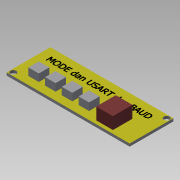
# Autodesk Inventor part: mode
Saved by Autodesk Inventor 2015 SP1 (Build 190203100, 203)
## iProperties
Created: 2015-01-28
Part Number: mode
Material: Generic
Document SubType Name: Modeling
Designer: Rafi Kurnia Putra
Density: 1 g/cm^3
Appearance: Default
Author: Rafi Kurnia Putra
Autodesk Inventor part; units mm, degrees
ref_plane "YZ Plane" through (0, 0, 0) normal (1, 0, 0) x (0, 1, 0)
ref_plane "XZ Plane" through (0, 0, 0) normal (0, 1, 0) x (-1, 0, 0)
ref_plane "XY Plane" through (0, 0, 0) normal (0, 0, 1) x (1, 0, 0)
sketch "Sketch1" plane through (0, 0, 0) normal (0, 1, 0) x (-1, 0, 0)
  line L0 (36.775, 13.07) -> (-36.775, 13.07)
  line L1 (-36.775, 13.07) -> (-36.775, -13.07)
  line L2 (-36.775, -13.07) -> (36.775, -13.07)
  line L3 (36.775, -13.07) -> (36.775, 13.07)
  line L4 (36.775, 13.07) -> (-36.775, -13.07) construction
  line L5 (-36.775, 13.07) -> (36.775, -13.07) construction
  circle A0 centre (-34.775, -11.07) radius 1.75
  circle A1 centre (34.775, 11.07) radius 1.75
  line L6 (-14.775, -0.61) -> (-24.775, -0.61)
  line L7 (-24.775, -0.61) -> (-24.775, 11.07)
  line L8 (-24.775, 11.07) -> (-14.775, 11.07)
  line L9 (-14.775, 11.07) -> (-14.775, -0.61)
  line L10 (-14.775, -0.61) -> (-24.775, 11.07) construction
  line L11 (-24.775, -0.61) -> (-14.775, 11.07) construction
  line L12 (28.4695, 2.1) -> (22.2095, 2.1)
  line L13 (22.2095, 2.1) -> (22.2095, 8.36)
  line L14 (22.2095, 8.36) -> (28.4695, 8.36)
  line L15 (28.4695, 8.36) -> (28.4695, 2.1)
  line L16 (28.4695, 2.1) -> (22.2095, 8.36) construction
  line L17 (22.2095, 2.1) -> (28.4695, 8.36) construction
  line L18 (18.4695, 8.36) -> (12.2095, 8.36)
  line L19 (12.2095, 8.36) -> (12.2095, 2.1)
  line L20 (12.2095, 2.1) -> (18.4695, 2.1)
  line L21 (18.4695, 2.1) -> (18.4695, 8.36)
  line L22 (18.4695, 8.36) -> (12.2095, 2.1) construction
  line L23 (12.2095, 8.36) -> (18.4695, 2.1) construction
  line L24 (8.4695, 8.36) -> (2.2095, 8.36)
  line L25 (2.2095, 8.36) -> (2.2095, 2.1)
  line L26 (2.2095, 2.1) -> (8.4695, 2.1)
  line L27 (8.4695, 2.1) -> (8.4695, 8.36)
  line L28 (8.4695, 8.36) -> (2.2095, 2.1) construction
  line L29 (2.2095, 8.36) -> (8.4695, 2.1) construction
  line L30 (-1.5305, 8.36) -> (-7.7905, 8.36)
  line L31 (-7.7905, 8.36) -> (-7.7905, 2.1)
  line L32 (-7.7905, 2.1) -> (-1.5305, 2.1)
  line L33 (-1.5305, 2.1) -> (-1.5305, 8.36)
  line L34 (-1.5305, 8.36) -> (-7.7905, 2.1) construction
  line L35 (-7.7905, 8.36) -> (-1.5305, 2.1) construction
  point P0 (0, 0)
  point P1 (-19.775, 5.23)
  point P2 (25.3395, 5.23)
  point P3 (15.3395, 5.23)
  point P4 (5.3395, 5.23)
  point P5 (-4.6605, 5.23)
  dimension "d0" = 73.55
  dimension "d1" = 26.14
  dimension "d2" = 3.5
  dimension "d3" = 2
  dimension "d4" = 2
  dimension "d5" = 3.5
  dimension "d6" = 2
  dimension "d7" = 2
  dimension "d8" = 10
  dimension "d9" = 11.68
  dimension "d10" = 12
  dimension "d11" = 2
  dimension "d12" = 6.26
  dimension "d13" = 6.26
  dimension "d14" = 6.26
  dimension "d15" = 6.26
  dimension "d16" = 10
  dimension "d17" = 6.26
  dimension "d18" = 6.26
  dimension "d19" = 10
  dimension "d20" = 6.26
  dimension "d21" = 6.26
  dimension "d22" = 10
  dimension "d23" = 6.9845
  constraints: 72 end point, 12 midpoint, 12 parallel, 6 horizontal, 6 perpendicular, 2 centre point
  measures "d0" distance of L2.end L1.end
  measures "d1" distance of L1.end L0.end
  measures "d2" diameter of A0
  measures "d3" distance from line of A0.centre L1
  measures "d4" distance from line of A0.centre L2
  measures "d5" diameter of A1
  measures "d6" distance from line of A1.centre L3
  measures "d7" distance from line of A1.centre L0
  measures "d8" distance of L7.end L8.end
  measures "d9" distance of L6.end L7.end
  measures "d10" distance between parallel lines of L1 L7
  measures "d11" distance between parallel lines of L0 L8
  measures "d12" distance of L13.end L14.end
  measures "d13" distance of L12.end L13.end
  measures "d14" distance of L20.end L19.end
  measures "d15" distance of L19.end L18.end
  measures "d16" distance of point (15.34, 5.23) point (25.34, 5.23)
  measures "d17" distance of L26.end L25.end
  measures "d18" distance of L25.end L24.end
  measures "d19" distance of point (5.34, 5.23) point (15.34, 5.23)
  measures "d20" distance of L32.end L31.end
  measures "d21" distance of L31.end L30.end
  measures "d22" distance of point (-4.66, 5.23) point (5.34, 5.23)
  measures "d23" distance between parallel lines of L9 L31
extrude "Extrusion1" add sketch "Sketch1" along normal blind 1.6
extrude "Extrusion2" add sketch "Sketch1" along normal blind 8.76 contours L6 L7 L8 L9
extrude "Extrusion3" add sketch "Sketch1" along normal blind 6 contours L12 L13 L14 L15 | L21 L20 L19 L18 | L27 L26 L25 L24 | L33 L32 L31 L30
sketch "Sketch2" plane through (0, 1.6, 0) normal (0, 1, 0) x (1, 0, 0)
  line L0 (-31.8499, 8.687) -> (29.6525, 8.687) construction
  line L1 (29.6525, 8.687) -> (29.6525, 4.9573) construction
  line L2 (29.6525, 4.9573) -> (-31.8499, 4.9573) construction
  line L3 (-31.8499, 4.9573) -> (-31.8499, 8.687) construction
  point P0 (0, 0)
  constraints: 2 other
body "Solid1"
